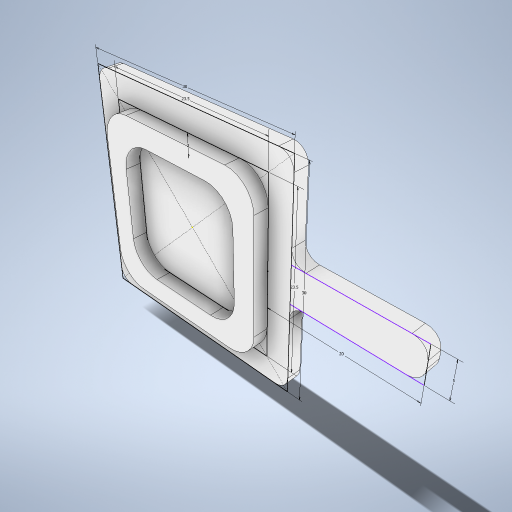
# Autodesk Inventor part: DustCover
Saved by Autodesk Inventor 2023 (Build 270158000, 158)
## iProperties
Created: 2022-10-01
Part Number: DustCover
Material: ABS Plastic
Document SubType Name: Modeling
Designer: Miner
Density: 1.06 g/cm^3
Appearance: Smooth - White
Author: Miner
Autodesk Inventor part; units mm, degrees
ref_plane "YZ Plane" through (0, 0, 0) normal (1, 0, 0) x (0, 1, 0)
ref_plane "XZ Plane" through (0, 0, 0) normal (0, 1, 0) x (-1, 0, 0)
ref_plane "XY Plane" through (0, 0, 0) normal (0, 0, 1) x (1, 0, 0)
sketch "Sketch1" plane through (0, 0, 0) normal (0, 0, 1) x (1, 0, 0)
  line L0 (-15, -15) -> (15, -15)
  line L1 (15, -15) -> (15, 15)
  line L2 (15, 15) -> (-15, 15)
  line L3 (-15, 15) -> (-15, -15)
  line L4 (-15, -15) -> (15, 15) construction
  line L5 (15, -15) -> (-15, 15) construction
  line L6 (-11.75, -11.75) -> (11.75, -11.75)
  line L7 (11.75, -11.75) -> (11.75, 11.75)
  line L8 (11.75, 11.75) -> (-11.75, 11.75)
  line L9 (-11.75, 11.75) -> (-11.75, -11.75)
  line L10 (-11.75, -11.75) -> (11.75, 11.75) construction
  line L11 (11.75, -11.75) -> (-11.75, 11.75) construction
  line L12 (-8.75, 8.75) -> (8.75, 8.75)
  line L13 (8.75, 8.75) -> (8.75, -8.75)
  line L14 (8.75, -8.75) -> (-8.75, -8.75)
  line L15 (-8.75, -8.75) -> (-8.75, 8.75)
  line L16 (15, -2.5) -> (31.75, -2.5)
  line L17 (31.75, -2.5) -> (31.75, 2.5)
  line L18 (31.75, 2.5) -> (15, 2.5)
  line L19 (15, 2.5) -> (15, -2.5)
  point P0 (0, 0)
  point P1 (11.75, 0)
  dimension "d0" = 30
  dimension "d1" = 30
  dimension "d2" = 23.5
  dimension "d3" = 23.5
  dimension "d4" = 3
  dimension "d10" = 5
  dimension "d12" = 20
  constraints: 40 end point, 8 parallel, 5 midpoint, 5 perpendicular, 2 horizontal, 1 point on line, 3 other
  measures "d0" distance of L2.end L1.end
  measures "d1" distance of L1.end L0.end
  measures "d2" distance of L8.end L7.end
  measures "d3" distance of L7.end L6.end
  measures "d4" distance between parallel lines of L8 L12
  measures "d10" distance of L17.end L16.end
  measures "d12" distance from line of point (11.75, 0) L17
extrude "Extrusion2" add sketch "Sketch1" against normal blind 2 contours L3 L2 L1 L0 | L9 L8 L7 L6 | L12 L13 L14 L15
extrude "Extrusion3" add sketch "Sketch1" against normal blind 2 contours L1 L18 L17 L16
fillet "Fillet2" radius 2 4 edges at (-15, -15, -1) (-15, 15, -1) (15, -15, -1) (15, 15, -1)
fillet "Fillet3" radius 2 4 edges at (31.75, -2.5, -1) (31.75, 2.5, -1) (15, 2.5, -1) (15, -2.5, -1)
extrude "Extrusion4" add sketch "Sketch1" along normal blind 2 contours L9 L8 L7 L6
fillet "Fillet4" radius 4 8 edges at (11.75, 11.75, 1) (11.75, -11.75, 1) (-11.75, -11.75, 1) (-11.75, 11.75, 1) (8.75, 8.75, 1) (-8.75, 8.75, 1) (-8.75, -8.75, 1) (8.75, -8.75, 1)
body "Solid1"
